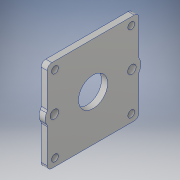
# Autodesk Inventor part: Intake Motor Mount
Saved by Autodesk Inventor 2019.4 (Build 234330000, 330)
## iProperties
Created: 2020-01-12
Part Number: Intake Motor Mount
Material: Aluminum 6061
Document SubType Name: Modeling
Designer: admin
Density: 2.7 g/cm^3
Appearance: Aluminum - Flat
Mass: 24.0624 g
Surface Area: 58.7968 cm^2
Volume: 8.91198 cm^3
Author: admin
Autodesk Inventor part; units mm, degrees
ref_plane "YZ Plane" through (0, 0, 0) normal (1, 0, 0) x (0, 1, 0)
ref_plane "XZ Plane" through (0, 0, 0) normal (0, 1, 0) x (-1, 0, 0)
ref_plane "XY Plane" through (0, 0, 0) normal (0, 0, 1) x (1, 0, 0)
sketch "Sketch1" plane through (0, 0, 0) normal (1, 0, 0) x (0, 1, 0)
  line L0 (-30, 30) -> (30, 30)
  line L1 (30, 30) -> (30, -30)
  line L2 (30, -30) -> (-30, -30)
  line L3 (-30, -30) -> (-30, 30)
  line L4 (-30, 30) -> (30, -30) construction
  line L5 (30, 30) -> (-30, -30) construction
  line L6 (-25, 25) -> (25, 25) construction
  line L7 (25, 25) -> (25, -25) construction
  line L8 (25, -25) -> (-25, -25) construction
  line L9 (-25, -25) -> (-25, 25) construction
  line L10 (-25, 25) -> (25, -25) construction
  line L11 (25, 25) -> (-25, -25) construction
  circle A0 centre (-25, 25) radius 2.2
  circle A1 centre (-25, -25) radius 2.2
  circle A2 centre (25, -25) radius 2.2
  circle A3 centre (25, 25) radius 2.2
  circle A4 centre (0, 0) radius 9.5
  line L12 (0, 25.4) -> (0, -25.4) construction
  circle A5 centre (0, 25.4) radius 6
  circle A6 centre (0, -25.4) radius 6
  circle A7 centre (0, -25.4) radius 2.75
  circle A8 centre (0, 25.4) radius 2.75
  point P0 (0, 0)
  point P1 (0, 0)
  dimension "d0" = 60
  dimension "d1" = 50
  dimension "d2" = 4.4
  dimension "d3" = 4.4
  dimension "d4" = 4.4
  dimension "d5" = 4.4
  dimension "d6" = 19
  dimension "d7" = 50.8
  dimension "d8" = 12
  dimension "d9" = 12
  dimension "d10" = 5.5
  dimension "d11" = 5.5
  constraints: 26 end point, 9 centre point, 9 coincident, 8 midpoint, 4 parallel, 3 perpendicular, 2 horizontal, 1 point on line, 1 vertical
  measures "d0" distance of L0.end L1.end
  measures "d1" distance of L6.end L7.end
  measures "d2" diameter of A0
  measures "d3" diameter of A1
  measures "d4" diameter of A2
  measures "d5" diameter of A3
  measures "d6" diameter of A4
  measures "d7" distance of L12.start L12.end
  measures "d8" diameter of A5
  measures "d9" diameter of A6
  measures "d10" diameter of A7
  measures "d11" diameter of A8
extrude "Extrusion1" add sketch "Sketch1" along normal blind 4
sketch "Sketch2" plane through (4, 0, 0) normal (1, 0, 0) x (0, 0, -1)
  arc A0 (-25, 2.7208) -> (-25, -2.7208) centre (-25.4, 0) ccw projected
  arc A1 (25, -2.7208) -> (25, 2.7208) centre (25.4, 0) ccw projected
  point P0 (0, 0)
  point P1 (-25.4, 0)
  point P2 (25.4, 0)
  constraints: 2 coincident
hole "Hole1" at (4, 0, 25.4) at (4, 0, -25.4) direction (-1, 0, 0) diameter 5.5 end through all
fillet "Fillet1" radius 3 8 edges at (2, 30, 30) (2, 30, -30) (2, -30, 30) (2, -30, -30) (2, 3.8523, 30) (2, -3.8523, 30) (2, -3.8523, -30) (2, 3.8523, -30)
body "Solid1"
